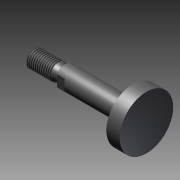
# Autodesk Inventor part: 536267 ADN-15-P-A_(KS)
Saved by Autodesk Inventor 2011 SP1 (Build 150282100, 282)
## iProperties
Created: 2018-05-26
Part Number: 536267 ADN-15-P-A_(KS)
Catalog Web Link: www.cadenas.de
Description: ADN-(KS)-Compact cylinder - piston rod
Vendor: FESTO
Document SubType Name: Modeling
Designer: psAdmin
Manufacturer: FESTO
Mass: 12.3954 g
Surface Area: 45.2592 cm^2
Volume: 12.3954 cm^3
Density: 1 g/cm^3
Category: PARTsolutions
Company: FESTO
Title: 536267 ADN-15-P-A_(KS)
Author: Cadenas PARTsolutions
Comments: Compact cylinder - piston rod
PSOL_IDENT_0: {$CADENAS_DATA\23d-libs\festo\parts\a\adn\parts\adn_ks.prj},229 {VTYP=3D},{NB=536267 ADN-15-P-A_(KS)
PSOL_IDENT_1: },{LINA=536267 ADN-15-P-A_(KS)},{NN=ADN-(KS)},{DATE=06.10.2015 11:54:02},{GEOMDATE=23.09.2015 12:10:
PSOL_IDENT_2: 00},{VERSION=},{LINEID=8220},{LINESUBID=-1},{WBVAR=DF,HUB,TH,Q,S2S20,K2,K5,K8,K10,S1,TT,R8}  {NB=536
PSOL_IDENT_3: 267 ADN-15-P-A_(KS)},{LINA=536267 ADN-15-P-A_(KS)},{KT=536267},{TNR=536267},{AUSF=ADN},{DF=P},{GA=A}
PSOL_IDENT_4: ,{WHX=6},{WH0=6.000},{WH1=0.000},{WH2=12.500},{WH3=6.500},{WHX1=6},{WHX2=6.75},{WH=6},{ZM=57.500},{Z
PSOL_IDENT_5: M2=58.600},{ZB=50.000},{ZB1=0.000},{ZB2=50.600},{ZB6=56.500},{ZA=44.000},{KDM=32},{HUBP=-},{HUB=15},
PSOL_IDENT_6: {HUB1=[1-400]},{HUB2=[1-300]},{HUB3=0},{HUB4=[1-400]},{TH=A},{THC='A','I'},{Q=-},{VAR1C='-','Q'},{S2
PSOL_IDENT_7: S20=-},{VAR2C='-','S2','S20'},{VAR22C='-','S2'},{VAR222C='-','S2','S20'},{K2=0},{VAR3C=0,[1-20]},{VA
PSOL_IDENT_8: R33C=0,[1-20]},{K5=-},{K5A='-','M10','M12'},{K5I='-','M6'},{K5S1A='-'},{K5S1I='-'},{K5C='-','M10','M
PSOL_IDENT_9: 12'},{K5N=0},{K5P=0},{K5T=},{K8=0},{K10=-},{K10A='-','K10'},{K10N=},{S1=-},{TT=-},{TT1='-','TT'},{R8=
PSOL_IDENT_10: -},{R81='-','R8'},{VAR4C=0,[1-400]},{VAR5C='-','S6'},{VAR6C='-'},{VAR66C='-'},{VAR7C='-','R3'},{HUBA
PSOL_IDENT_11: LG=[1-400]},{A=19.000},{A1=0.000},{AF=16.000},{AF1=0.000},{AF2=14.000},{AF3=0.000},{AF5=14.000},{AF7=
PSOL_IDENT_12: 0.000},{D8=4.500},{D9=8.000},{KF=M8},{KFN=8.000},{KF1=-},{KF1C=0.0000},{KF2=-},{KF2C=0.0000},{KF3=M6
PSOL_IDENT_13: },{KF3C=6.0000},{KF5=M6},{KF5N=6},{KF7=-},{KF7N=0},{KK=M10X1.25},{KKN=10},{KKP=1.25},{KK1=-},{KK1N=0
PSOL_IDENT_14: .0000},{KK1P=0.00},{L2=44.000},{L8=3.000},{MM=12.000},{MM1=0.000},{PL=8.200},{SF=10},{SF1=0},{SF3=10
PSOL_IDENT_15: .0},{WL=4.700},{WL1=0.000},{QN=},{S2N=},{S1N=},{K2N=},{K8N=},{KKC3=8.200},{KKF2=0.600},{KKD5=1.500},
PSOL_IDENT_16: {KKE2=20.000},{K5C3=0},{K5F2=0},{K5D5=0},{KK1C3=0.000},{KK1F2=0.000},{KK1D5=0.000},{KK1E2=0.000},{L1
PSOL_IDENT_17: 00S1=0.000},{L101S1=0.000},{L102S1=0.000},{L103S1=0.000},{D100S1=0.000},{L100=0.600},{L101=3.300},{L
PSOL_IDENT_18: 102=16.000},{L103=20.000},{D100=8.400},{L100Q=0.400},{L101Q=2.600},{L101K5=2.600},{L102Q=14.000},{L1
PSOL_IDENT_19: 03Q=18.000},{D100Q=6.400},{L100S1K5=0.000},{L101S1K5=0.000},{L102S1K5=0.000},{L103S1K5=0.000},{D100S
PSOL_IDENT_20: 1K5=0.000},{VERS=2},{TTN=},{R8N=},{D20=0.000},{XF31=4.000},{B31=5.000},{DFALG='P','PPS'}
NN: ADN-(KS)
NT: Compact cylinder - piston rod
NB: 536267 ADN-15-P-A_(KS)
NBSYN: $TNR. $AUSF.-$HUB.-$DF.-$TH.$QN.$S2N.$K2N.$K5T.$K8N.$K10N.$S1N.$TTN.$R8N._(KS)
LINA: 536267 ADN-15-P-A_(KS)
TNR: 536267
AUSF: ADN
DF: P
GA: A
WHX: 6.000
WH0: 6.000
WH1: 0.000
WH2: 12.500
WH3: 6.500
WHX1: 6.000
WHX2: 6.750
WH: 6.000
ZM: 57.500
ZM2: 58.600
ZB: 50.000
ZB1: 0.000
ZB2: 50.600
ZB6: 56.500
ZA: 44.000
KDM: 32
HUBP: -
HUB: 15
TH: A
Q: -
S2S20: -
K2: 0
K5: -
K8: 0
K10: -
S1: -
TT: -
R8: -
A: 19.000
A1: 0.000
AF: 16.000
AF1: 0.000
AF2: 14.000
AF3: 0.000
AF5: 14.000
AF7: 0.000
D8: 4.500
D9: 8.000
KF: M8
KF1: -
KF2: -
KF3: M6
KF5: M6
KF7: -
KK: M10X1.25
KK1: -
L2: 44.000
L8: 3.000
MM: 12.000
MM1: 0.000
PL: 8.200
SF: 10
SF1: 0
SF3: 10.0
WL: 4.700
WL1: 0.000
L101K5: 2.600
D20: 0.000
XF31: 4.000
B31: 5.000
SUPPLIER: FESTO
ARTICLENO: 536267 ADN-15-P-A_(KS)
BOMINFO: 536267 ADN-15-P-A_(KS)
CREATOR: CADENAS GmbH
Autodesk Inventor part; units mm, degrees
sketch "Sketch_1" plane through (0, 0, 0) normal (0, 0, 1) x (1, 0, 0)
  line L0 (42.6, 0) -> (-6, 0)
  line L1 (-6, 0) -> (-6, 6)
  line L2 (-6, 6) -> (42.6, 6)
  line L3 (42.6, 6) -> (42.6, 0)
  line L4 (42.6, 0) -> (-6, 0)
  constraints: 10 end point
revolve "Revolution1" add sketch "Sketch_1" angle 360 about axis through (42.6, 0, 0) along (1, 0, 0)
sketch "Sketch_11" plane through (0, 0, 0) normal (0, 0, 1) x (1, 0, 0)
  line L0 (42.6, 0) -> (34.6, 0)
  line L1 (34.6, 0) -> (34.6, 16)
  line L2 (34.6, 16) -> (42.6, 16)
  line L3 (42.6, 16) -> (42.6, 0)
  line L4 (42.6, 0) -> (34.6, 0)
  constraints: 10 end point
revolve "Revolution2" add sketch "Sketch_11" angle 360 about axis through (42.6, 0, 0) along (1, 0, 0)
sketch "Sketch_19" plane through (0, 0, 0) normal (0, 0, 1) x (1, 0, 0)
  line L0 (-5, 0) -> (-25, 0)
  line L1 (-25, 0) -> (-25, 4.233)
  line L2 (-25, 4.233) -> (-24.233, 5)
  line L3 (-24.233, 5) -> (-9.9727, 5)
  line L4 (-9.9727, 5) -> (-7.5994, 4.1362)
  arc A0 (-7.5994, 4.1362) -> (-7.3942, 4.1) centre (-7.3942, 4.7) ccw
  line L5 (-7.3942, 4.1) -> (-6.6, 4.1)
  arc A1 (-6.6, 4.1) -> (-6, 4.7) centre (-6.6, 4.7) ccw
  line L6 (-6, 4.7) -> (-6, 5)
  line L7 (-6, 5) -> (-5, 5)
  line L8 (-5, 5) -> (-5, 0)
  line L9 (-5, 0) -> (-25, 0)
  constraints: 20 end point, 4 point on circle, 2 centre point
revolve "Revolution3" add sketch "Sketch_19" angle 360 about axis through (-5, 0, 0) along (1, 0, 0)
thread "Thread1" size "M10x1.25" class "6g" standard "ISO Metric profile" full length
sketch "Sketch_20" plane through (0, 0, 0) normal (0, 0, 1) x (1, 0, 0)
  line L0 (-36, -16) -> (5.0509, -16)
  line L1 (5.0509, -16) -> (-1.3, -5)
  line L2 (-1.3, -5) -> (-6, -5)
  line L3 (-6, -5) -> (-6, -10)
  line L4 (-6, -10) -> (-30, -10)
  line L5 (-30, -10) -> (-30, 10)
  line L6 (-30, 10) -> (-6, 10)
  line L7 (-6, 10) -> (-6, 5)
  line L8 (-6, 5) -> (-1.3, 5)
  line L9 (-1.3, 5) -> (5.0509, 16)
  line L10 (5.0509, 16) -> (-36, 16)
  line L11 (-36, 16) -> (-36, -16)
  constraints: 24 end point
extrude "Extrusion1" cut sketch "Sketch_20" along normal mid plane 24
ref_plane "FDT_PIRODACC_M1_XY" through (-15, 0, 0) normal (-1, 0, 0) x (0, 1, 0)
ref_plane "FDT_PIRODACC_M1_YZ" through (-15, 0, 0) normal (0, 1, 0) x (0, 0, -1)
ref_plane "FDT_PIRODACC_M1_ZX" through (-15, 0, 0) normal (0, 0, -1) x (-1, 0, 0)
ref_plane "NUT1_XY" through (-12.5, 0, 0) normal (1, 0, 0) x (0, 0, -1)
ref_plane "NUT1_YZ" through (-12.5, 0, 0) normal (0, 0, -1) x (0, 1, 0)
ref_plane "NUT1_ZX" through (-12.5, 0, 0) normal (0, 1, 0) x (1, 0, 0)
ref_plane "PISTON_XY" through (42.6, 0, 0) normal (1, 0, 0) x (0, 0, -1)
ref_plane "PISTON_YZ" through (42.6, 0, 0) normal (0, 0, -1) x (0, 1, 0)
ref_plane "PISTON_ZX" through (42.6, 0, 0) normal (0, 1, 0) x (1, 0, 0)
body "Solid1"
